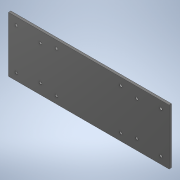
# Autodesk Inventor part: Power Distribution Board - Chassis redo
Saved by Autodesk Inventor 2020.2 (Build 242310000, 310)
## iProperties
Created: 2020-08-21
Part Number: Power Distribution Board - Chassis redo
Material: Generic
Document SubType Name: Modeling
Designer: Krishna Makhija
Density: 1 g/cm^3
Appearance: Default
Author: Krishna Makhija
Autodesk Inventor part; units mm, degrees
ref_plane "YZ Plane" through (0, 0, 0) normal (1, 0, 0) x (0, 1, 0)
ref_plane "XZ Plane" through (0, 0, 0) normal (0, 1, 0) x (-1, 0, 0)
ref_plane "XY Plane" through (0, 0, 0) normal (0, 0, 1) x (1, 0, 0)
sketch "Sketch1" plane through (0, 0, 0) normal (0, 0, 1) x (1, 0, 0)
  line L0 (-100, 34.4999) -> (100, 34.4999)
  line L1 (100, 34.4999) -> (100, -34.4999)
  line L2 (100, -34.4999) -> (-100, -34.4999)
  line L3 (-100, -34.4999) -> (-100, 34.4999)
  line L4 (-100, 34.4999) -> (100, -34.4999) construction
  line L5 (100, 34.4999) -> (-100, -34.4999) construction
  circle A0 centre (40, 25.5) radius 1.5
  line L6 (-40, 55.9999) -> (160, -12.9999) construction
  line L7 (160, 55.9999) -> (-40, -12.9999) construction
  circle A1 centre (60, 21.5) radius 1.5
  circle A2 centre (90, 25.5) radius 1.5
  circle A3 centre (-40, -25.5) radius 1.5
  circle A4 centre (40, -25.5) radius 1.5
  circle A5 centre (-40, 25.5) radius 1.5
  circle A6 centre (-60, -21.5) radius 1.5
  circle A7 centre (-60, 21.5) radius 1.5
  circle A8 centre (60, -21.5) radius 1.5
  circle A9 centre (90, -25.5) radius 1.5
  circle A10 centre (-90, -25.5) radius 1.5
  circle A11 centre (-90, 25.5) radius 1.5
  constraints: 16 end point, 12 centre point, 2 parallel, 1 horizontal, 1 perpendicular
extrude "Extrusion1" add sketch "Sketch1" along normal blind 3
body "Solid1"
